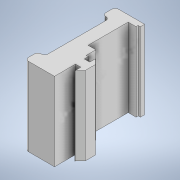
# Autodesk Inventor part: Tape_Belt_Layer
Saved by Autodesk Inventor 2021 (Build 250183000, 183)
## iProperties
Created: 2021-08-10
Part Number: Tape_Belt_Layer
Material: Generic
Document SubType Name: Modeling
Designer: Jorian Brusind
Density: 1 g/cm^3
Appearance: Default
Author: Jorian Brusind
Autodesk Inventor part; units mm, degrees
ref_plane "YZ Plane" through (0, 0, 0) normal (1, 0, 0) x (0, 1, 0)
ref_plane "XZ Plane" through (0, 0, 0) normal (0, 1, 0) x (-1, 0, 0)
ref_plane "XY Plane" through (0, 0, 0) normal (0, 0, 1) x (1, 0, 0)
sketch "Sketch1" plane through (0, 0, 0) normal (0, 1, 0) x (-1, 0, 0)
  line L0 (-7.5, -23) -> (7.5, -23)
  line L1 (7.5, -23) -> (7.5, 23)
  line L2 (7.5, 23) -> (-7.5, 23)
  line L3 (-7.5, 23) -> (-7.5, -23)
  line L4 (-7.5, -23) -> (7.5, 23) construction
  line L5 (7.5, -23) -> (-7.5, 23) construction
  point P0 (0, 0)
  dimension "d0" = 15
  dimension "d1" = 46
  constraints: 12 end point, 2 midpoint, 2 parallel, 1 horizontal, 1 perpendicular
  measures "d0" distance of L2.end L1.end
  measures "d1" distance of L1.end L0.end
extrude "Extrusion1" add sketch "Sketch1" along normal blind 40
sketch "Sketch2" plane through (0, 40, 0) normal (0, 1, 0) x (1, 0, 0)
  line L0 (7.5, -23) -> (7.5, 23) projected
  line L1 (7.5, 23) -> (-7.5, 23) projected
  line L2 (7.5, 23) -> (6.9285, 23)
  line L3 (6.9285, 23) -> (6.9285, 7.3)
  line L4 (6.357, 20.3) -> (7.5, 20.3)
  line L5 (7.5, 20.3) -> (7.5, -5.7)
  line L6 (7.5, -5.7) -> (6.357, -5.7)
  line L7 (6.357, -5.7) -> (6.357, 20.3)
  line L8 (6.357, 20.3) -> (7.5, -5.7) construction
  line L9 (7.5, 20.3) -> (6.357, -5.7) construction
  point P0 (7.5, -5.7)
  point P1 (7.5, 20.3)
  dimension "d7" = 0.5715
  dimension "d8" = 15.7
  dimension "d9" = 90
  dimension "d10" = 1.143
  dimension "d11" = 26
  constraints: 16 end point, 2 midpoint, 2 parallel, 2 perpendicular, 1 horizontal, 1 point on line
  measures "d7" distance of L0.end L2.end
  measures "d8" distance of L2.end L3.end
  measures "d9" angle of L3 L2
  measures "d10" distance of L5.end L6.end
  measures "d11" distance of L4.end L5.end
extrude "Extrusion2" cut sketch "Sketch2" against normal through all contours L6 L7 L4 L0
sketch "Sketch3" plane through (0, 40, 0) normal (0, 1, 0) x (1, 0, 0)
  line L0 (6.357, -5.7) -> (6.357, 20.3) projected
  line L1 (5.357, 9.5) -> (4.357, 9.5)
  line L2 (2.357, 19.75) -> (6.357, 19.75)
  line L3 (6.357, 19.75) -> (6.357, -0.75)
  line L4 (6.357, -0.75) -> (2.357, -0.75)
  line L5 (2.357, -0.75) -> (2.357, 19.75)
  line L6 (2.357, 19.75) -> (6.357, -0.75) construction
  line L7 (6.357, 19.75) -> (2.357, -0.75) construction
  line L8 (7.5, 23) -> (-7.5, 23) projected
  point P0 (6.357, -0.75)
  point P1 (6.357, 19.75)
  dimension "d51" = 1
  dimension "d53" = 4
  dimension "d54" = 20.5
  dimension "d59" = 4
  dimension "d60" = 90
  dimension "d61" = 13.5
  constraints: 14 end point, 2 midpoint, 2 parallel, 1 horizontal, 1 perpendicular
  measures "d51" distance of L1.start L1.end
  measures "d53" distance of L3.end L4.end
  measures "d54" distance of L2.end L3.end
  measures "d59" distance between parallel lines of L0 L5
  measures "d60" angle of L0 L1
  measures "d61" distance from line of L8 L1.end
sketch "Sketch4" plane through (0, 40, 0) normal (0, 1, 0) x (1, 0, 0)
  line L0 (7.5, -23) -> (7.5, -5.7) projected
  line L1 (7.5, -23) -> (7.5, -10)
  line L2 (7.5, -10) -> (9.5, -10)
  line L3 (9.5, -10) -> (9.5, -16)
  line L4 (9.5, -10) -> (9.5, -4)
  line L5 (9.5, -10) -> (13.5, -10)
  line L6 (13.5, -10) -> (13.5, -12.9395)
  line L7 (13.5, -10) -> (13.5, -7.06)
  line L8 (9.5, -16) -> (10.439, -16)
  line L9 (9.5, -4) -> (10.439, -4)
  line L10 (10.439, -4) -> (13.5, -7.06)
  line L11 (13.5, -12.9395) -> (10.439, -16)
  line L12 (9.5, -10) -> (9.5, -13)
  line L13 (9.5, -10) -> (9.5, -7)
  line L14 (9.5, -10) -> (12.5, -10) construction
  line L15 (9.5, -7) -> (7.5, -7)
  line L16 (9.5, -13) -> (7.5, -13)
  line L17 (7.5, -13) -> (7.5, -7)
  line L18 (10.25, -10.95) -> (10.25, -15.25)
  line L19 (10.25, -15.25) -> (10.1284, -15.25)
  line L20 (10.1284, -15.25) -> (12.75, -12.6288)
  line L21 (12.75, -12.6288) -> (12.75, -13)
  line L22 (12.75, -13) -> (12.75, -7.3707)
  line L23 (12.75, -7.3707) -> (10.1284, -4.75)
  line L24 (10.1284, -4.75) -> (10.25, -4.75)
  line L25 (10.25, -4.75) -> (10.25, -10.25)
  line L26 (10.25, -13.1) -> (12.45, -13.1) construction
  line L27 (10.25, -7.5) -> (12.15, -7.5) construction
  line L28 (7.5, -23) -> (7.5, -5.7) projected
  line L29 (10.25, -10.95) -> (10.25, -10.25)
  line L30 (8.5, -13) -> (8.5, -12.25)
  line L31 (8.5, -12.25) -> (10.25, -12.25)
  line L32 (8.5, -12.25) -> (7.5, -12.25)
  line L33 (8.5, -7) -> (8.5, -7.75)
  line L34 (8.5, -7.75) -> (7.5, -7.75)
  line L35 (8.5, -7.75) -> (10.25, -7.75)
  point P0 (0, 0)
  point P1 (9.5, -7)
  point P2 (7.5, -7)
  point P3 (9.5, -7.1)
  point P4 (10.25, -10)
  point P5 (12.75, -10)
  point P6 (10.25, -13)
  point P7 (7.75, -10.75)
  point P8 (10.25, -4.8715)
  point P9 (10.25, -15.1284)
  dimension "d19" = 13
  dimension "d20" = 2
  dimension "d21" = 6
  dimension "d22" = 6
  dimension "d23" = 4
  dimension "d24" = 2.9395
  dimension "d25" = 2.94
  dimension "d26" = 0.939
  dimension "d27" = 0.939
  dimension "d28" = 3
  dimension "d29" = 3
  dimension "d30" = 90
  dimension "d31" = 0.75
  dimension "d32" = 0.75
  dimension "d47" = 0.75
  dimension "d48" = 0.75
  constraints: 68 end point, 9 point on line, 7 horizontal, 7 perpendicular, 5 midpoint, 4 vertical, 2 collinear, 6 other
  measures "d19" distance of L0.start L1.end
  measures "d20" distance of L1.end L2.end
  measures "d21" distance of L2.end L3.end
  measures "d22" distance of L2.end L4.end
  measures "d23" distance of L2.end L5.end
  measures "d24" distance of L5.end L6.end
  measures "d25" distance of L5.end L7.end
  measures "d26" distance of L3.end L8.end
  measures "d27" distance of L4.end L9.end
  measures "d28" distance of L2.end L12.end
  measures "d29" distance of L2.end L13.end
  measures "d30" angle of L14 L13
  measures "d31" distance between parallel lines of L11 L20
  measures "d32" distance between parallel lines of L10 L23
  measures "d47" distance of L30.start L30.end
  measures "d48" distance of L33.start L33.end
extrude "Extrusion5" add sketch "Sketch4" against normal up to surface (40 mm away) contours L0 L2 L3 L31 L32 | L0 L34 L35 L4 L2 | L18 L19 L20 | L5 L25 L29 L18 L31 L3 | L4 L35 L25 L5 | L25 L23 L22 L5 | L5 L22 L20 L18 L29 L25
sketch "Sketch5" plane through (0, 40, 0) normal (0, 1, 0) x (1, 0, 0)
  line L0 (-11, 16.5) -> (-4, 16.5)
  line L1 (-4, 16.5) -> (-4, -16.5)
  line L2 (-4, -16.5) -> (-11, -16.5)
  line L3 (-11, -16.5) -> (-11, 16.5)
  line L4 (-7.5, 23) -> (-7.5, -23) projected
  line L5 (-11, 16.5) -> (-4, -16.5) construction
  line L6 (-4, 16.5) -> (-11, -16.5) construction
  point P0 (0, 0)
  point P1 (-7.5, 0)
  point P2 (-7.5, 16.5)
  point P3 (-7.5, -16.5)
  dimension "d41" = 7
  dimension "d42" = 33
  constraints: 12 end point, 3 midpoint, 2 parallel, 1 horizontal, 1 perpendicular
  measures "d41" distance of L1.end L2.end
  measures "d42" distance of L0.end L1.end
extrude "Extrusion6" cut sketch "Sketch5" against normal through all contours L0 L1 L2 L4
fillet "Fillet1" radius 1.75 4 edges at (-7.5, 20, 16.5) (-7.5, 20, 23) (-7.5, 20, -16.5) (-7.5, 20, -23)
fillet "Fillet2" radius 1.75 2 edges at (-4, 20, -16.5) (-4, 20, 16.5)
move faces "Move3" translate (0, 0, -0.5) faces at (7.119, 26.6667, -20.3)
extrude "Extrusion7" cut sketch "Sketch3" against normal through all
body "Solid1"
